Autodesk Inventor part; units mm, degrees
(part 2 of 2)
  line L899 (32.6279, -72.4956) -> (36.6693, -72.5044)
  line L900 (30.5996, -75.9912) -> (32.6279, -72.4956)
  line L901 (32.6127, -79.4956) -> (30.5996, -75.9912)
  line L902 (36.6541, -79.5044) -> (32.6127, -79.4956)
  line L903 (-30.5996, 19.9912) -> (-32.6279, 16.4956)
  line L904 (-32.6127, 23.4956) -> (-30.5996, 19.9912)
  line L905 (-36.6541, 23.5044) -> (-32.6127, 23.4956)
  line L906 (-38.6825, 20.0088) -> (-36.6541, 23.5044)
  line L907 (-36.6693, 16.5044) -> (-38.6825, 20.0088)
  line L908 (-32.6279, 16.4956) -> (-36.6693, 16.5044)
  line L909 (-30.5996, 27.9912) -> (-32.6279, 24.4956)
  line L910 (-32.6127, 31.4956) -> (-30.5996, 27.9912)
  line L911 (-36.6541, 31.5044) -> (-32.6127, 31.4956)
  line L912 (-38.6825, 28.0088) -> (-36.6541, 31.5044)
  line L913 (-36.6693, 24.5044) -> (-38.6825, 28.0088)
  line L914 (-32.6279, 24.4956) -> (-36.6693, 24.5044)
  line L915 (-30.5996, 11.9912) -> (-32.6279, 8.4956)
  line L916 (-32.6127, 15.4956) -> (-30.5996, 11.9912)
  line L917 (-36.6541, 15.5044) -> (-32.6127, 15.4956)
  line L918 (-38.6825, 12.0088) -> (-36.6541, 15.5044)
  line L919 (-36.6693, 8.5044) -> (-38.6825, 12.0088)
  line L920 (-32.6279, 8.4956) -> (-36.6693, 8.5044)
  line L921 (-30.5996, 35.9912) -> (-32.6279, 32.4956)
  line L922 (-32.6127, 39.4956) -> (-30.5996, 35.9912)
  line L923 (-36.6541, 39.5044) -> (-32.6127, 39.4956)
  line L924 (-38.6825, 36.0088) -> (-36.6541, 39.5044)
  line L925 (-36.6693, 32.5044) -> (-38.6825, 36.0088)
  line L926 (-32.6279, 32.4956) -> (-36.6693, 32.5044)
  line L927 (-30.5996, 3.9912) -> (-32.6279, 0.4956)
  line L928 (-32.6127, 7.4956) -> (-30.5996, 3.9912)
  line L929 (-36.6541, 7.5044) -> (-32.6127, 7.4956)
  line L930 (-38.6825, 4.0088) -> (-36.6541, 7.5044)
  line L931 (-36.6693, 0.5044) -> (-38.6825, 4.0088)
  line L932 (-32.6279, 0.4956) -> (-36.6693, 0.5044)
  line L933 (-30.5996, 43.9912) -> (-32.6279, 40.4956)
  line L934 (-32.6127, 47.4956) -> (-30.5996, 43.9912)
  line L935 (-36.6541, 47.5044) -> (-32.6127, 47.4956)
  line L936 (-38.6825, 44.0088) -> (-36.6541, 47.5044)
  line L937 (-36.6693, 40.5044) -> (-38.6825, 44.0088)
  line L938 (-32.6279, 40.4956) -> (-36.6693, 40.5044)
  line L939 (-30.5996, -4.0088) -> (-32.6279, -7.5044)
  line L940 (-32.6127, -0.5044) -> (-30.5996, -4.0088)
  line L941 (-36.6541, -0.4956) -> (-32.6127, -0.5044)
  line L942 (-38.6825, -3.9912) -> (-36.6541, -0.4956)
  line L943 (-36.6693, -7.4956) -> (-38.6825, -3.9912)
  line L944 (-32.6279, -7.5044) -> (-36.6693, -7.4956)
  line L945 (-30.5996, 51.9912) -> (-32.6279, 48.4956)
  line L946 (-32.6127, 55.4956) -> (-30.5996, 51.9912)
  line L947 (-36.6541, 55.5044) -> (-32.6127, 55.4956)
  line L948 (-38.6825, 52.0088) -> (-36.6541, 55.5044)
  line L949 (-36.6693, 48.5044) -> (-38.6825, 52.0088)
  line L950 (-32.6279, 48.4956) -> (-36.6693, 48.5044)
  line L951 (-30.5996, -12.0088) -> (-32.6279, -15.5044)
  line L952 (-32.6127, -8.5044) -> (-30.5996, -12.0088)
  line L953 (-36.6541, -8.4956) -> (-32.6127, -8.5044)
  line L954 (-38.6825, -11.9912) -> (-36.6541, -8.4956)
  line L955 (-36.6693, -15.4956) -> (-38.6825, -11.9912)
  line L956 (-32.6279, -15.5044) -> (-36.6693, -15.4956)
  line L957 (-30.5996, 59.9912) -> (-32.6279, 56.4956)
  line L958 (-32.6127, 63.4956) -> (-30.5996, 59.9912)
  line L959 (-36.6541, 63.5044) -> (-32.6127, 63.4956)
  line L960 (-38.6825, 60.0088) -> (-36.6541, 63.5044)
  line L961 (-36.6693, 56.5044) -> (-38.6825, 60.0088)
  line L962 (-32.6279, 56.4956) -> (-36.6693, 56.5044)
  line L963 (-30.5996, -20.0088) -> (-32.6279, -23.5044)
  line L964 (-32.6127, -16.5044) -> (-30.5996, -20.0088)
  line L965 (-36.6541, -16.4956) -> (-32.6127, -16.5044)
  line L966 (-38.6825, -19.9912) -> (-36.6541, -16.4956)
  line L967 (-36.6693, -23.4956) -> (-38.6825, -19.9912)
  line L968 (-32.6279, -23.5044) -> (-36.6693, -23.4956)
  line L969 (-30.5996, 67.9912) -> (-32.6279, 64.4956)
  line L970 (-32.6127, 71.4956) -> (-30.5996, 67.9912)
  line L971 (-36.6541, 71.5044) -> (-32.6127, 71.4956)
  line L972 (-38.6825, 68.0088) -> (-36.6541, 71.5044)
  line L973 (-36.6693, 64.5044) -> (-38.6825, 68.0088)
  line L974 (-32.6279, 64.4956) -> (-36.6693, 64.5044)
  line L975 (-30.5996, -28.0088) -> (-32.6279, -31.5044)
  line L976 (-32.6127, -24.5044) -> (-30.5996, -28.0088)
  line L977 (-36.6541, -24.4956) -> (-32.6127, -24.5044)
  line L978 (-38.6825, -27.9912) -> (-36.6541, -24.4956)
  line L979 (-36.6693, -31.4956) -> (-38.6825, -27.9912)
  line L980 (-32.6279, -31.5044) -> (-36.6693, -31.4956)
  line L981 (-30.5996, 75.9912) -> (-32.6279, 72.4956)
  line L982 (-32.6127, 79.4956) -> (-30.5996, 75.9912)
  line L983 (-36.6541, 79.5044) -> (-32.6127, 79.4956)
  line L984 (-38.6825, 76.0088) -> (-36.6541, 79.5044)
  line L985 (-36.6693, 72.5044) -> (-38.6825, 76.0088)
  line L986 (-32.6279, 72.4956) -> (-36.6693, 72.5044)
  line L987 (-30.5996, -36.0088) -> (-32.6279, -39.5044)
  line L988 (-32.6127, -32.5044) -> (-30.5996, -36.0088)
  line L989 (-36.6541, -32.4956) -> (-32.6127, -32.5044)
  line L990 (-38.6825, -35.9912) -> (-36.6541, -32.4956)
  line L991 (-36.6693, -39.4956) -> (-38.6825, -35.9912)
  line L992 (-32.6279, -39.5044) -> (-36.6693, -39.4956)
  line L993 (45.6107, -24.0088) -> (43.5823, -27.5044)
  line L994 (43.5975, -20.5044) -> (45.6107, -24.0088)
  line L995 (39.5561, -20.4956) -> (43.5975, -20.5044)
  line L996 (37.5278, -23.9912) -> (39.5561, -20.4956)
  line L997 (39.5409, -27.4956) -> (37.5278, -23.9912)
  line L998 (43.5823, -27.5044) -> (39.5409, -27.4956) construction
  line L999 (45.6107, -16.0088) -> (43.5823, -19.5044)
  line L1000 (43.5975, -12.5044) -> (45.6107, -16.0088)
  line L1001 (39.5561, -12.4956) -> (43.5975, -12.5044)
  line L1002 (37.5278, -15.9912) -> (39.5561, -12.4956)
  line L1003 (39.5409, -19.4956) -> (37.5278, -15.9912)
  line L1004 (43.5823, -19.5044) -> (39.5409, -19.4956)
  line L1005 (45.6107, -32.0088) -> (43.5823, -35.5044)
  line L1006 (43.5975, -28.5044) -> (45.6107, -32.0088)
  line L1007 (39.5561, -28.4956) -> (43.5975, -28.5044)
  line L1008 (37.5278, -31.9912) -> (39.5561, -28.4956)
  line L1009 (39.5409, -35.4956) -> (37.5278, -31.9912)
  line L1010 (43.5823, -35.5044) -> (39.5409, -35.4956)
  line L1011 (45.6107, -8.0088) -> (43.5823, -11.5044)
  line L1012 (43.5975, -4.5044) -> (45.6107, -8.0088)
  line L1013 (39.5561, -4.4956) -> (43.5975, -4.5044)
  line L1014 (37.5278, -7.9912) -> (39.5561, -4.4956)
  line L1015 (39.5409, -11.4956) -> (37.5278, -7.9912)
  line L1016 (43.5823, -11.5044) -> (39.5409, -11.4956)
  line L1017 (45.6107, -40.0088) -> (43.5823, -43.5044)
  line L1018 (43.5975, -36.5044) -> (45.6107, -40.0088)
  line L1019 (39.5561, -36.4956) -> (43.5975, -36.5044)
  line L1020 (37.5278, -39.9912) -> (39.5561, -36.4956)
  line L1021 (39.5409, -43.4956) -> (37.5278, -39.9912)
  line L1022 (43.5823, -43.5044) -> (39.5409, -43.4956)
  line L1023 (45.6107, -0.0088) -> (43.5823, -3.5044)
  line L1024 (43.5975, 3.4956) -> (45.6107, -0.0088)
  line L1025 (39.5561, 3.5044) -> (43.5975, 3.4956)
  line L1026 (37.5278, 0.0088) -> (39.5561, 3.5044)
  line L1027 (39.5409, -3.4956) -> (37.5278, 0.0088)
  line L1028 (43.5823, -3.5044) -> (39.5409, -3.4956)
  line L1029 (45.6107, -48.0088) -> (43.5823, -51.5044)
  line L1030 (43.5975, -44.5044) -> (45.6107, -48.0088)
  line L1031 (39.5561, -44.4956) -> (43.5975, -44.5044)
  line L1032 (37.5278, -47.9912) -> (39.5561, -44.4956)
  line L1033 (39.5409, -51.4956) -> (37.5278, -47.9912)
  line L1034 (43.5823, -51.5044) -> (39.5409, -51.4956)
  line L1035 (45.6107, 7.9912) -> (43.5823, 4.4956)
  line L1036 (43.5975, 11.4956) -> (45.6107, 7.9912)
  line L1037 (39.5561, 11.5044) -> (43.5975, 11.4956)
  line L1038 (37.5278, 8.0088) -> (39.5561, 11.5044)
  line L1039 (39.5409, 4.5044) -> (37.5278, 8.0088)
  line L1040 (43.5823, 4.4956) -> (39.5409, 4.5044)
  line L1041 (45.6107, -56.0088) -> (43.5823, -59.5044)
  line L1042 (43.5975, -52.5044) -> (45.6107, -56.0088)
  line L1043 (39.5561, -52.4956) -> (43.5975, -52.5044)
  line L1044 (37.5278, -55.9912) -> (39.5561, -52.4956)
  line L1045 (39.5409, -59.4956) -> (37.5278, -55.9912)
  line L1046 (43.5823, -59.5044) -> (39.5409, -59.4956)
  line L1047 (45.6107, 15.9912) -> (43.5823, 12.4956)
  line L1048 (43.5975, 19.4956) -> (45.6107, 15.9912)
  line L1049 (39.5561, 19.5044) -> (43.5975, 19.4956)
  line L1050 (37.5278, 16.0088) -> (39.5561, 19.5044)
  line L1051 (39.5409, 12.5044) -> (37.5278, 16.0088)
  line L1052 (43.5823, 12.4956) -> (39.5409, 12.5044)
  line L1053 (45.6107, -64.0088) -> (43.5823, -67.5044)
  line L1054 (43.5975, -60.5044) -> (45.6107, -64.0088)
  line L1055 (39.5561, -60.4956) -> (43.5975, -60.5044)
  line L1056 (37.5278, -63.9912) -> (39.5561, -60.4956)
  line L1057 (39.5409, -67.4956) -> (37.5278, -63.9912)
  line L1058 (43.5823, -67.5044) -> (39.5409, -67.4956)
  line L1059 (45.6107, 23.9912) -> (43.5823, 20.4956)
  line L1060 (43.5975, 27.4956) -> (45.6107, 23.9912)
  line L1061 (39.5561, 27.5044) -> (43.5975, 27.4956)
  line L1062 (37.5278, 24.0088) -> (39.5561, 27.5044)
  line L1063 (39.5409, 20.5044) -> (37.5278, 24.0088)
  line L1064 (43.5823, 20.4956) -> (39.5409, 20.5044)
  line L1065 (45.6107, -72.0088) -> (43.5823, -75.5044)
  line L1066 (43.5975, -68.5044) -> (45.6107, -72.0088)
  line L1067 (39.5561, -68.4956) -> (43.5975, -68.5044)
  line L1068 (37.5278, -71.9912) -> (39.5561, -68.4956)
  line L1069 (39.5409, -75.4956) -> (37.5278, -71.9912)
  line L1070 (43.5823, -75.5044) -> (39.5409, -75.4956)
  line L1071 (45.6107, 31.9912) -> (43.5823, 28.4956)
  line L1072 (43.5975, 35.4956) -> (45.6107, 31.9912)
  line L1073 (39.5561, 35.5044) -> (43.5975, 35.4956)
  line L1074 (37.5278, 32.0088) -> (39.5561, 35.5044)
  line L1075 (39.5409, 28.5044) -> (37.5278, 32.0088)
  line L1076 (43.5823, 28.4956) -> (39.5409, 28.5044)
  line L1077 (45.6107, -80.0088) -> (43.5823, -83.5044)
  line L1078 (43.5975, -76.5044) -> (45.6107, -80.0088)
  line L1079 (39.5561, -76.4956) -> (43.5975, -76.5044)
  line L1080 (37.5278, -79.9912) -> (39.5561, -76.4956)
  line L1081 (39.5409, -83.4956) -> (37.5278, -79.9912)
  line L1082 (43.5823, -83.5044) -> (39.5409, -83.4956)
  line L1083 (-37.5278, 23.9912) -> (-39.5561, 20.4956)
  line L1084 (-39.5409, 27.4956) -> (-37.5278, 23.9912)
  line L1085 (-43.5823, 27.5044) -> (-39.5409, 27.4956)
  line L1086 (-45.6107, 24.0088) -> (-43.5823, 27.5044)
  line L1087 (-43.5975, 20.5044) -> (-45.6107, 24.0088)
  line L1088 (-39.5561, 20.4956) -> (-43.5975, 20.5044)
  line L1089 (-37.5278, 31.9912) -> (-39.5561, 28.4956)
  line L1090 (-39.5409, 35.4956) -> (-37.5278, 31.9912)
  line L1091 (-43.5823, 35.5044) -> (-39.5409, 35.4956)
  line L1092 (-45.6107, 32.0088) -> (-43.5823, 35.5044)
  line L1093 (-43.5975, 28.5044) -> (-45.6107, 32.0088)
  line L1094 (-39.5561, 28.4956) -> (-43.5975, 28.5044)
  line L1095 (-37.5278, 15.9912) -> (-39.5561, 12.4956)
  line L1096 (-39.5409, 19.4956) -> (-37.5278, 15.9912)
  line L1097 (-43.5823, 19.5044) -> (-39.5409, 19.4956)
  line L1098 (-45.6107, 16.0088) -> (-43.5823, 19.5044)
  line L1099 (-43.5975, 12.5044) -> (-45.6107, 16.0088)
  line L1100 (-39.5561, 12.4956) -> (-43.5975, 12.5044)
  line L1101 (-37.5278, 39.9912) -> (-39.5561, 36.4956)
  line L1102 (-39.5409, 43.4956) -> (-37.5278, 39.9912)
  line L1103 (-43.5823, 43.5044) -> (-39.5409, 43.4956)
  line L1104 (-45.6107, 40.0088) -> (-43.5823, 43.5044)
  line L1105 (-43.5975, 36.5044) -> (-45.6107, 40.0088)
  line L1106 (-39.5561, 36.4956) -> (-43.5975, 36.5044)
  line L1107 (-37.5278, 7.9912) -> (-39.5561, 4.4956)
  line L1108 (-39.5409, 11.4956) -> (-37.5278, 7.9912)
  line L1109 (-43.5823, 11.5044) -> (-39.5409, 11.4956)
  line L1110 (-45.6107, 8.0088) -> (-43.5823, 11.5044)
  line L1111 (-43.5975, 4.5044) -> (-45.6107, 8.0088)
  line L1112 (-39.5561, 4.4956) -> (-43.5975, 4.5044)
  line L1113 (-37.5278, 47.9912) -> (-39.5561, 44.4956)
  line L1114 (-39.5409, 51.4956) -> (-37.5278, 47.9912)
  line L1115 (-43.5823, 51.5044) -> (-39.5409, 51.4956)
  line L1116 (-45.6107, 48.0088) -> (-43.5823, 51.5044)
  line L1117 (-43.5975, 44.5044) -> (-45.6107, 48.0088)
  line L1118 (-39.5561, 44.4956) -> (-43.5975, 44.5044)
  line L1119 (-37.5278, -0.0088) -> (-39.5561, -3.5044)
  line L1120 (-39.5409, 3.4956) -> (-37.5278, -0.0088)
  line L1121 (-43.5823, 3.5044) -> (-39.5409, 3.4956)
  line L1122 (-45.6107, 0.0088) -> (-43.5823, 3.5044)
  line L1123 (-43.5975, -3.4956) -> (-45.6107, 0.0088)
  line L1124 (-39.5561, -3.5044) -> (-43.5975, -3.4956)
  line L1125 (-37.5278, 55.9912) -> (-39.5561, 52.4956)
  line L1126 (-39.5409, 59.4956) -> (-37.5278, 55.9912)
  line L1127 (-43.5823, 59.5044) -> (-39.5409, 59.4956)
  line L1128 (-45.6107, 56.0088) -> (-43.5823, 59.5044)
  line L1129 (-43.5975, 52.5044) -> (-45.6107, 56.0088)
  line L1130 (-39.5561, 52.4956) -> (-43.5975, 52.5044)
  line L1131 (-37.5278, -8.0088) -> (-39.5561, -11.5044)
  line L1132 (-39.5409, -4.5044) -> (-37.5278, -8.0088)
  line L1133 (-43.5823, -4.4956) -> (-39.5409, -4.5044)
  line L1134 (-45.6107, -7.9912) -> (-43.5823, -4.4956)
  line L1135 (-43.5975, -11.4956) -> (-45.6107, -7.9912)
  line L1136 (-39.5561, -11.5044) -> (-43.5975, -11.4956)
  line L1137 (-37.5278, 63.9912) -> (-39.5561, 60.4956)
  line L1138 (-39.5409, 67.4956) -> (-37.5278, 63.9912)
  line L1139 (-43.5823, 67.5044) -> (-39.5409, 67.4956)
  line L1140 (-45.6107, 64.0088) -> (-43.5823, 67.5044)
  line L1141 (-43.5975, 60.5044) -> (-45.6107, 64.0088)
  line L1142 (-39.5561, 60.4956) -> (-43.5975, 60.5044)
  line L1143 (-37.5278, -16.0088) -> (-39.5561, -19.5044)
  line L1144 (-39.5409, -12.5044) -> (-37.5278, -16.0088)
  line L1145 (-43.5823, -12.4956) -> (-39.5409, -12.5044)
  line L1146 (-45.6107, -15.9912) -> (-43.5823, -12.4956)
  line L1147 (-43.5975, -19.4956) -> (-45.6107, -15.9912)
  line L1148 (-39.5561, -19.5044) -> (-43.5975, -19.4956)
  line L1149 (-37.5278, 71.9912) -> (-39.5561, 68.4956)
  line L1150 (-39.5409, 75.4956) -> (-37.5278, 71.9912)
  line L1151 (-43.5823, 75.5044) -> (-39.5409, 75.4956)
  line L1152 (-45.6107, 72.0088) -> (-43.5823, 75.5044)
  line L1153 (-43.5975, 68.5044) -> (-45.6107, 72.0088)
  line L1154 (-39.5561, 68.4956) -> (-43.5975, 68.5044)
  line L1155 (-37.5278, -24.0088) -> (-39.5561, -27.5044)
  line L1156 (-39.5409, -20.5044) -> (-37.5278, -24.0088)
  line L1157 (-43.5823, -20.4956) -> (-39.5409, -20.5044)
  line L1158 (-45.6107, -23.9912) -> (-43.5823, -20.4956)
  line L1159 (-43.5975, -27.4956) -> (-45.6107, -23.9912)
  line L1160 (-39.5561, -27.5044) -> (-43.5975, -27.4956)
  line L1161 (-37.5278, 79.9912) -> (-39.5561, 76.4956)
  line L1162 (-39.5409, 83.4956) -> (-37.5278, 79.9912)
  line L1163 (-43.5823, 83.5044) -> (-39.5409, 83.4956)
  line L1164 (-45.6107, 80.0088) -> (-43.5823, 83.5044)
  line L1165 (-43.5975, 76.5044) -> (-45.6107, 80.0088)
  line L1166 (-39.5561, 76.4956) -> (-43.5975, 76.5044)
  line L1167 (-37.5278, -32.0088) -> (-39.5561, -35.5044)
  line L1168 (-39.5409, -28.5044) -> (-37.5278, -32.0088)
  line L1169 (-43.5823, -28.4956) -> (-39.5409, -28.5044)
  line L1170 (-45.6107, -31.9912) -> (-43.5823, -28.4956)
  line L1171 (-43.5975, -35.4956) -> (-45.6107, -31.9912)
  line L1172 (-39.5561, -35.5044) -> (-43.5975, -35.4956)
  line L1173 (52.5389, -28.0088) -> (50.5105, -31.5044)
  line L1174 (50.5257, -24.5044) -> (52.5389, -28.0088)
  line L1175 (46.4843, -24.4956) -> (50.5257, -24.5044)
  line L1176 (44.456, -27.9912) -> (46.4843, -24.4956)
  line L1177 (46.4691, -31.4956) -> (44.456, -27.9912)
  line L1178 (50.5105, -31.5044) -> (46.4691, -31.4956)
  line L1179 (52.5389, -20.0088) -> (50.5105, -23.5044) construction
  line L1180 (50.5257, -16.5044) -> (52.5389, -20.0088) construction
  line L1181 (46.4843, -16.4956) -> (50.5257, -16.5044)
  line L1182 (44.456, -19.9912) -> (46.4843, -16.4956)
  line L1183 (46.4691, -23.4956) -> (44.456, -19.9912)
  line L1184 (50.5105, -23.5044) -> (46.4691, -23.4956)
  line L1185 (52.5389, -36.0088) -> (50.5105, -39.5044)
  line L1186 (50.5257, -32.5044) -> (52.5389, -36.0088)
  line L1187 (46.4843, -32.4956) -> (50.5257, -32.5044)
  line L1188 (44.456, -35.9912) -> (46.4843, -32.4956)
  line L1189 (46.4691, -39.4956) -> (44.456, -35.9912)
  line L1190 (50.5105, -39.5044) -> (46.4691, -39.4956)
  line L1191 (52.5389, -12.0088) -> (50.5105, -15.5044)
  line L1192 (50.5257, -8.5044) -> (52.5389, -12.0088)
  line L1193 (46.4843, -8.4956) -> (50.5257, -8.5044)
  line L1194 (44.456, -11.9912) -> (46.4843, -8.4956)
  line L1195 (46.4691, -15.4956) -> (44.456, -11.9912)
  line L1196 (50.5105, -15.5044) -> (46.4691, -15.4956)
  line L1197 (52.5389, -44.0088) -> (50.5105, -47.5044)
  line L1198 (50.5257, -40.5044) -> (52.5389, -44.0088)
  line L1199 (46.4843, -40.4956) -> (50.5257, -40.5044)
  line L1200 (44.456, -43.9912) -> (46.4843, -40.4956)
  line L1201 (46.4691, -47.4956) -> (44.456, -43.9912)
  line L1202 (50.5105, -47.5044) -> (46.4691, -47.4956)
  line L1203 (52.5389, -4.0088) -> (50.5105, -7.5044)
  line L1204 (50.5257, -0.5044) -> (52.5389, -4.0088)
  line L1205 (46.4843, -0.4956) -> (50.5257, -0.5044)
  line L1206 (44.456, -3.9912) -> (46.4843, -0.4956)
  line L1207 (46.4691, -7.4956) -> (44.456, -3.9912)
  line L1208 (50.5105, -7.5044) -> (46.4691, -7.4956)
  line L1209 (52.5389, -52.0088) -> (50.5105, -55.5044)
  line L1210 (50.5257, -48.5044) -> (52.5389, -52.0088)
  line L1211 (46.4843, -48.4956) -> (50.5257, -48.5044)
  line L1212 (44.456, -51.9912) -> (46.4843, -48.4956)
  line L1213 (46.4691, -55.4956) -> (44.456, -51.9912)
  line L1214 (50.5105, -55.5044) -> (46.4691, -55.4956)
  line L1215 (52.5389, 3.9912) -> (50.5105, 0.4956)
  line L1216 (50.5257, 7.4956) -> (52.5389, 3.9912)
  line L1217 (46.4843, 7.5044) -> (50.5257, 7.4956)
  line L1218 (44.456, 4.0088) -> (46.4843, 7.5044)
  line L1219 (46.4691, 0.5044) -> (44.456, 4.0088)
  line L1220 (50.5105, 0.4956) -> (46.4691, 0.5044)
  line L1221 (52.5389, -60.0088) -> (50.5105, -63.5044)
  line L1222 (50.5257, -56.5044) -> (52.5389, -60.0088)
  line L1223 (46.4843, -56.4956) -> (50.5257, -56.5044)
  line L1224 (44.456, -59.9912) -> (46.4843, -56.4956)
  line L1225 (46.4691, -63.4956) -> (44.456, -59.9912)
  line L1226 (50.5105, -63.5044) -> (46.4691, -63.4956)
  line L1227 (52.5389, 11.9912) -> (50.5105, 8.4956)
  line L1228 (50.5257, 15.4956) -> (52.5389, 11.9912)
  line L1229 (46.4843, 15.5044) -> (50.5257, 15.4956)
  line L1230 (44.456, 12.0088) -> (46.4843, 15.5044)
  line L1231 (46.4691, 8.5044) -> (44.456, 12.0088)
  line L1232 (50.5105, 8.4956) -> (46.4691, 8.5044)
  line L1233 (52.5389, -68.0088) -> (50.5105, -71.5044)
  line L1234 (50.5257, -64.5044) -> (52.5389, -68.0088)
  line L1235 (46.4843, -64.4956) -> (50.5257, -64.5044)
  line L1236 (44.456, -67.9912) -> (46.4843, -64.4956)
  line L1237 (46.4691, -71.4956) -> (44.456, -67.9912)
  line L1238 (50.5105, -71.5044) -> (46.4691, -71.4956)
  line L1239 (52.5389, 19.9912) -> (50.5105, 16.4956)
  line L1240 (50.5257, 23.4956) -> (52.5389, 19.9912)
  line L1241 (46.4843, 23.5044) -> (50.5257, 23.4956)
  line L1242 (44.456, 20.0088) -> (46.4843, 23.5044)
  line L1243 (46.4691, 16.5044) -> (44.456, 20.0088)
  line L1244 (50.5105, 16.4956) -> (46.4691, 16.5044)
  line L1245 (52.5389, -76.0088) -> (50.5105, -79.5044)
  line L1246 (50.5257, -72.5044) -> (52.5389, -76.0088)
  line L1247 (46.4843, -72.4956) -> (50.5257, -72.5044)
  line L1248 (44.456, -75.9912) -> (46.4843, -72.4956)
  line L1249 (46.4691, -79.4956) -> (44.456, -75.9912)
  line L1250 (50.5105, -79.5044) -> (46.4691, -79.4956)
  line L1251 (52.5389, 27.9912) -> (50.5105, 24.4956)
  line L1252 (50.5257, 31.4956) -> (52.5389, 27.9912)
  line L1253 (46.4843, 31.5044) -> (50.5257, 31.4956)
  line L1254 (44.456, 28.0088) -> (46.4843, 31.5044)
  line L1255 (46.4691, 24.5044) -> (44.456, 28.0088)
  line L1256 (50.5105, 24.4956) -> (46.4691, 24.5044)
  line L1257 (52.5389, -84.0088) -> (50.5105, -87.5044)
  line L1258 (50.5257, -80.5044) -> (52.5389, -84.0088)
  line L1259 (46.4843, -80.4956) -> (50.5257, -80.5044)
  line L1260 (44.456, -83.9912) -> (46.4843, -80.4956)
  line L1261 (46.4691, -87.4956) -> (44.456, -83.9912)
  line L1262 (50.5105, -87.5044) -> (46.4691, -87.4956)
  line L1263 (-44.456, 27.9912) -> (-46.4843, 24.4956)
  line L1264 (-46.4691, 31.4956) -> (-44.456, 27.9912)
  line L1265 (-50.5105, 31.5044) -> (-46.4691, 31.4956)
  line L1266 (-52.5389, 28.0088) -> (-50.5105, 31.5044)
  line L1267 (-50.5257, 24.5044) -> (-52.5389, 28.0088)
  line L1268 (-46.4843, 24.4956) -> (-50.5257, 24.5044)
  line L1269 (-44.456, 35.9912) -> (-46.4843, 32.4956)
  line L1270 (-46.4691, 39.4956) -> (-44.456, 35.9912)
  line L1271 (-50.5105, 39.5044) -> (-46.4691, 39.4956)
  line L1272 (-52.5389, 36.0088) -> (-50.5105, 39.5044)
  line L1273 (-50.5257, 32.5044) -> (-52.5389, 36.0088)
  line L1274 (-46.4843, 32.4956) -> (-50.5257, 32.5044)
  line L1275 (-44.456, 19.9912) -> (-46.4843, 16.4956)
  line L1276 (-46.4691, 23.4956) -> (-44.456, 19.9912)
  line L1277 (-50.5105, 23.5044) -> (-46.4691, 23.4956)
  line L1278 (-52.5389, 20.0088) -> (-50.5105, 23.5044)
  line L1279 (-50.5257, 16.5044) -> (-52.5389, 20.0088)
  line L1280 (-46.4843, 16.4956) -> (-50.5257, 16.5044)
  line L1281 (-44.456, 43.9912) -> (-46.4843, 40.4956)
  line L1282 (-46.4691, 47.4956) -> (-44.456, 43.9912)
  line L1283 (-50.5105, 47.5044) -> (-46.4691, 47.4956)
  line L1284 (-52.5389, 44.0088) -> (-50.5105, 47.5044)
  line L1285 (-50.5257, 40.5044) -> (-52.5389, 44.0088)
  line L1286 (-46.4843, 40.4956) -> (-50.5257, 40.5044)
  line L1287 (-44.456, 11.9912) -> (-46.4843, 8.4956)
  line L1288 (-46.4691, 15.4956) -> (-44.456, 11.9912)
  line L1289 (-50.5105, 15.5044) -> (-46.4691, 15.4956)
  line L1290 (-52.5389, 12.0088) -> (-50.5105, 15.5044)
  line L1291 (-50.5257, 8.5044) -> (-52.5389, 12.0088)
  line L1292 (-46.4843, 8.4956) -> (-50.5257, 8.5044)
  line L1293 (-44.456, 51.9912) -> (-46.4843, 48.4956)
  line L1294 (-46.4691, 55.4956) -> (-44.456, 51.9912)
  line L1295 (-50.5105, 55.5044) -> (-46.4691, 55.4956)
  line L1296 (-52.5389, 52.0088) -> (-50.5105, 55.5044)
  line L1297 (-50.5257, 48.5044) -> (-52.5389, 52.0088)
  line L1298 (-46.4843, 48.4956) -> (-50.5257, 48.5044)
  line L1299 (-44.456, 3.9912) -> (-46.4843, 0.4956)
  line L1300 (-46.4691, 7.4956) -> (-44.456, 3.9912)
  line L1301 (-50.5105, 7.5044) -> (-46.4691, 7.4956)
  line L1302 (-52.5389, 4.0088) -> (-50.5105, 7.5044)
  line L1303 (-50.5257, 0.5044) -> (-52.5389, 4.0088)
  line L1304 (-46.4843, 0.4956) -> (-50.5257, 0.5044)
  line L1305 (-44.456, 59.9912) -> (-46.4843, 56.4956)
  line L1306 (-46.4691, 63.4956) -> (-44.456, 59.9912)
  line L1307 (-50.5105, 63.5044) -> (-46.4691, 63.4956)
  line L1308 (-52.5389, 60.0088) -> (-50.5105, 63.5044)
  line L1309 (-50.5257, 56.5044) -> (-52.5389, 60.0088)
  line L1310 (-46.4843, 56.4956) -> (-50.5257, 56.5044)
  line L1311 (-44.456, -4.0088) -> (-46.4843, -7.5044)
  line L1312 (-46.4691, -0.5044) -> (-44.456, -4.0088)
  line L1313 (-50.5105, -0.4956) -> (-46.4691, -0.5044)
  line L1314 (-52.5389, -3.9912) -> (-50.5105, -0.4956)
  line L1315 (-50.5257, -7.4956) -> (-52.5389, -3.9912)
  line L1316 (-46.4843, -7.5044) -> (-50.5257, -7.4956)
  line L1317 (-44.456, 67.9912) -> (-46.4843, 64.4956)
  line L1318 (-46.4691, 71.4956) -> (-44.456, 67.9912)
  line L1319 (-50.5105, 71.5044) -> (-46.4691, 71.4956)
  line L1320 (-52.5389, 68.0088) -> (-50.5105, 71.5044)
  line L1321 (-50.5257, 64.5044) -> (-52.5389, 68.0088)
  line L1322 (-46.4843, 64.4956) -> (-50.5257, 64.5044)
  line L1323 (-44.456, -12.0088) -> (-46.4843, -15.5044)
  line L1324 (-46.4691, -8.5044) -> (-44.456, -12.0088)
  line L1325 (-50.5105, -8.4956) -> (-46.4691, -8.5044)
  line L1326 (-52.5389, -11.9912) -> (-50.5105, -8.4956)
  line L1327 (-50.5257, -15.4956) -> (-52.5389, -11.9912)
  line L1328 (-46.4843, -15.5044) -> (-50.5257, -15.4956)
  line L1329 (-44.456, 75.9912) -> (-46.4843, 72.4956)
  line L1330 (-46.4691, 79.4956) -> (-44.456, 75.9912)
  line L1331 (-50.5105, 79.5044) -> (-46.4691, 79.4956)
  line L1332 (-52.5389, 76.0088) -> (-50.5105, 79.5044)
  line L1333 (-50.5257, 72.5044) -> (-52.5389, 76.0088)
  line L1334 (-46.4843, 72.4956) -> (-50.5257, 72.5044)
  line L1335 (-44.456, -20.0088) -> (-46.4843, -23.5044)
  line L1336 (-46.4691, -16.5044) -> (-44.456, -20.0088)
  line L1337 (-50.5105, -16.4956) -> (-46.4691, -16.5044)
  line L1338 (-52.5389, -19.9912) -> (-50.5105, -16.4956)
  line L1339 (-50.5257, -23.4956) -> (-52.5389, -19.9912)
  line L1340 (-46.4843, -23.5044) -> (-50.5257, -23.4956)
  line L1341 (-44.456, 83.9912) -> (-46.4843, 80.4956)
  line L1342 (-46.4691, 87.4956) -> (-44.456, 83.9912)
  line L1343 (-50.5105, 87.5044) -> (-46.4691, 87.4956)
  line L1344 (-52.5389, 84.0088) -> (-50.5105, 87.5044)
  line L1345 (-50.5257, 80.5044) -> (-52.5389, 84.0088)
  line L1346 (-46.4843, 80.4956) -> (-50.5257, 80.5044)
  line L1347 (-44.456, -28.0088) -> (-46.4843, -31.5044)
  line L1348 (-46.4691, -24.5044) -> (-44.456, -28.0088)
  line L1349 (-50.5105, -24.4956) -> (-46.4691, -24.5044)
  line L1350 (-52.5389, -27.9912) -> (-50.5105, -24.4956)
  line L1351 (-50.5257, -31.4956) -> (-52.5389, -27.9912)
  line L1352 (-46.4843, -31.5044) -> (-50.5257, -31.4956)
  circle A0 centre (0, 0) radius 47.5 projected
  circle A1 centre (0, 0) radius 46.5
  line L1353 (30.5996, 36.0088) -> (32.6127, 32.5044)
  line L1354 (32.6127, 32.5044) -> (36.6541, 32.4956)
  line L1355 (30.5996, 36.0088) -> (32.6279, 39.5044)
  line L1356 (46.4843, 15.5044) -> (44.456, 12.0088)
  line L1357 (46.4691, 8.5044) -> (50.5105, 8.4956)
  line L1358 (46.4691, 8.5044) -> (44.456, 12.0088)
  line L1359 (50.5257, -8.5044) -> (46.4843, -8.4956)
  line L1360 (44.456, -11.9912) -> (46.4691, -15.4956)
  line L1361 (46.4843, -8.4956) -> (44.456, -11.9912)
  line L1362 (36.6693, -32.5044) -> (32.6279, -32.4956)
  line L1363 (30.5996, -35.9912) -> (32.6127, -39.4956)
  line L1364 (32.6279, -32.4956) -> (30.5996, -35.9912)
  line L1365 (17.8978, -48.0088) -> (15.8847, -44.5044)
  line L1366 (11.8433, -44.4956) -> (15.8847, -44.5044)
  line L1367 (9.815, -47.9912) -> (11.8281, -51.4956)
  line L1368 (11.8433, -44.4956) -> (9.815, -47.9912)
  line L1369 (-11.8281, -44.5044) -> (-15.8695, -44.4956)
  line L1370 (-17.8978, -47.9912) -> (-15.8695, -44.4956)
  line L1371 (-11.8281, -44.5044) -> (-9.815, -48.0088)
  line L1372 (39.5409, -27.4956) -> (43.5823, -27.5044)
  circle A2 centre (0, 0) radius 52.5 projected
  point P0 (-0.0076, -3.5)
  point P1 (3.0311, 6.25)
  point P2 (0, 11.5)
  point P3 (-0.0076, 4.5)
  point P4 (3.0311, -9.75)
  point P5 (0, -4.5)
  point P6 (-0.0076, -11.5)
  point P7 (3.0311, 14.25)
  point P8 (0, 19.5)
  point P9 (-0.0076, 12.5)
  point P10 (3.0311, -17.75)
  point P11 (0, -12.5)
  point P12 (-0.0076, -19.5)
  point P13 (3.0311, 22.25)
  point P14 (0, 27.5)
  point P15 (-0.0076, 20.5)
  point P16 (3.0311, -25.75)
  point P17 (0, -20.5)
  point P18 (-0.0076, -27.5)
  point P19 (3.0311, 30.25)
  point P20 (0, 35.5)
  point P21 (-0.0076, 28.5)
  point P22 (3.0311, -33.75)
  point P23 (0, -28.5)
  point P24 (-0.0076, -35.5)
  point P25 (3.0311, 38.25)
  point P26 (0, 43.5)
  point P27 (-0.0076, 36.5)
  point P28 (3.0311, -41.75)
  point P29 (0, -36.5)
  point P30 (-0.0076, -43.5)
  point P31 (3.0311, 46.25)
  point P32 (0, 51.5)
  point P33 (-0.0076, 44.5)
  point P34 (3.0311, -49.75)
  point P35 (0, -44.5)
  point P36 (-0.0076, -51.5)
  point P37 (3.0311, 54.25)
  point P38 (0, 59.5)
  point P39 (-0.0076, 52.5)
  point P40 (3.0311, -57.75)
  point P41 (0, -52.5)
  point P42 (-0.0076, -59.5)
  point P43 (9.9593, -5.75)
  point P44 (6.9282, -0.5)
  point P45 (6.9206, -7.5)
  point P46 (9.9593, 2.25)
  point P47 (6.9282, 7.5)
  point P48 (6.9206, 0.5)
  point P49 (9.9593, -13.75)
  point P50 (6.9282, -8.5)
  point P51 (6.9206, -15.5)
  point P52 (9.9593, 10.25)
  point P53 (6.9282, 15.5)
  point P54 (6.9206, 8.5)
  point P55 (9.9593, -21.75)
  point P56 (6.9282, -16.5)
  point P57 (6.9206, -23.5)
  point P58 (9.9593, 18.25)
  point P59 (6.9282, 23.5)
  point P60 (6.9206, 16.5)
  point P61 (9.9593, -29.75)
  point P62 (6.9282, -24.5)
  point P63 (6.9206, -31.5)
  point P64 (9.9593, 26.25)
  point P65 (6.9282, 31.5)
  point P66 (6.9206, 24.5)
  point P67 (9.9593, -37.75)
  point P68 (6.9282, -32.5)
  point P69 (6.9206, -39.5)
  point P70 (9.9593, 34.25)
  point P71 (6.9282, 39.5)
  point P72 (6.9206, 32.5)
  point P73 (9.9593, -45.75)
  point P74 (6.9282, -40.5)
  point P75 (6.9206, -47.5)
  point P76 (9.9593, 42.25)
  point P77 (6.9282, 47.5)
  point P78 (6.9206, 40.5)
  point P79 (9.9593, -53.75)
  point P80 (6.9282, -48.5)
  point P81 (6.9206, -55.5)
  point P82 (9.9593, 50.25)
  point P83 (6.9282, 55.5)
  point P84 (6.9206, 48.5)
  point P85 (9.9593, -61.75)
  point P86 (6.9282, -56.5)
  point P87 (6.9206, -63.5)
  point P88 (-3.8971, 2.25)
  point P89 (-6.9282, 7.5)
  point P90 (-6.9358, 0.5)
  point P91 (-3.8971, 10.25)
  point P92 (-6.9282, 15.5)
  point P93 (-6.9358, 8.5)
  point P94 (-3.8971, -5.75)
  point P95 (-6.9282, -0.5)
  point P96 (-6.9358, -7.5)
  point P97 (-3.8971, 18.25)
  point P98 (-6.9282, 23.5)
  point P99 (-6.9358, 16.5)
  point P100 (-3.8971, -13.75)
  point P101 (-6.9282, -8.5)
  point P102 (-6.9358, -15.5)
  point P103 (-3.8971, 26.25)
  point P104 (-6.9282, 31.5)
  point P105 (-6.9358, 24.5)
  point P106 (-3.8971, -21.75)
  point P107 (-6.9282, -16.5)
  point P108 (-6.9358, -23.5)
  point P109 (-3.8971, 34.25)
  point P110 (-6.9282, 39.5)
  point P111 (-6.9358, 32.5)
  point P112 (-3.8971, -29.75)
  point P113 (-6.9282, -24.5)
  point P114 (-6.9358, -31.5)
  point P115 (-3.8971, 42.25)
  point P116 (-6.9282, 47.5)
  point P117 (-6.9358, 40.5)
  point P118 (-3.8971, -37.75)
  point P119 (-6.9282, -32.5)
  point P120 (-6.9358, -39.5)
  point P121 (-3.8971, 50.25)
  point P122 (-6.9282, 55.5)
  point P123 (-6.9358, 48.5)
  point P124 (-3.8971, -45.75)
  point P125 (-6.9282, -40.5)
  point P126 (-6.9358, -47.5)
  point P127 (-3.8971, 58.25)
  point P128 (-6.9282, 63.5)
  point P129 (-6.9358, 56.5)
  point P130 (-3.8971, -53.75)
  point P131 (-6.9282, -48.5)
  point P132 (-6.9358, -55.5)
  point P133 (16.8875, -9.75)
  point P134 (13.8564, -4.5)
  point P135 (13.8488, -11.5)
  point P136 (16.8875, -1.75)
  point P137 (13.8564, 3.5)
  point P138 (13.8488, -3.5)
  point P139 (16.8875, -17.75)
  point P140 (13.8564, -12.5)
  point P141 (13.8488, -19.5)
  point P142 (16.8875, 6.25)
  point P143 (13.8564, 11.5)
  point P144 (13.8488, 4.5)
  point P145 (16.8875, -25.75)
  point P146 (13.8564, -20.5)
  point P147 (13.8488, -27.5)
  point P148 (16.8875, 14.25)
  point P149 (13.8564, 19.5)
  point P150 (13.8488, 12.5)
  point P151 (16.8875, -33.75)
  point P152 (13.8564, -28.5)
  point P153 (13.8488, -35.5)
  point P154 (16.8875, 22.25)
  point P155 (13.8564, 27.5)
  point P156 (13.8488, 20.5)
  point P157 (16.8875, -41.75)
  point P158 (13.8564, -36.5)
  point P159 (13.8488, -43.5)
  point P160 (16.8875, 30.25)
  point P161 (13.8564, 35.5)
  point P162 (13.8488, 28.5)
  point P163 (16.8875, -49.75)
  point P164 (13.8564, -44.5)
  point P165 (13.8488, -51.5)
  point P166 (16.8875, 38.25)
  point P167 (13.8564, 43.5)
  point P168 (13.8488, 36.5)
  point P169 (16.8875, -57.75)
  point P170 (13.8564, -52.5)
  point P171 (13.8488, -59.5)
  point P172 (16.8875, 46.25)
  point P173 (13.8564, 51.5)
  point P174 (13.8488, 44.5)
  point P175 (16.8875, -65.75)
  point P176 (13.8564, -60.5)
  point P177 (13.8488, -67.5)
  point P178 (-10.8253, 6.25)
  point P179 (-13.8564, 11.5)
  point P180 (-13.864, 4.5)
  point P181 (-10.8253, 14.25)
  point P182 (-13.8564, 19.5)
  point P183 (-13.864, 12.5)
  point P184 (-10.8253, -1.75)
  point P185 (-13.8564, 3.5)
  point P186 (-13.864, -3.5)
  point P187 (-10.8253, 22.25)
  point P188 (-13.8564, 27.5)
  point P189 (-13.864, 20.5)
  point P190 (-10.8253, -9.75)
  point P191 (-13.8564, -4.5)
  point P192 (-13.864, -11.5)
  point P193 (-10.8253, 30.25)
  point P194 (-13.8564, 35.5)
  point P195 (-13.864, 28.5)
  point P196 (-10.8253, -17.75)
  point P197 (-13.8564, -12.5)
  point P198 (-13.864, -19.5)
  point P199 (-10.8253, 38.25)
  dimension "d65" = 7
  dimension "d69" = 8
  dimension "d72" = 8
  constraints: 2746 end point, 450 point on line, 20 equal length, 2 coincident, 1 horizontal, 1 midpoint, 1 perpendicular, 1 vertical, 3376 other
  measures "d65" distance from line of point (-0.008, -3.5) L2
  measures "d69" distance of L3.end L9.start
  measures "d72" distance of L3.end L93.start
extrude "Extrusion10" cut sketch "Sketch14" against normal blind 10 contours L21 L26 L25 L24 L23 L22 | L27 L32 L31 L30 L29 L28 | L33 L38 L37 L36 L35 L34 | L39 L44 L43 L42 L41 L40 | L45 L50 L49 L48 L47 L46 | L51 L56 L55 L54 L53 L52 | L57 L62 L61 L60 L59 L58 | L63 L68 L67 L66 L65 L64 | L69 L74 L73 A1 | A1 L160 L159 L164 L163 L162 | L238 L237 L242 L241 L240 A1 | A1 L356 L355 | L417 L422 A1 | A1 L531 L536 L535 | L585 L590 L589 A1 | A1 L716 L715 L714 | L754 L753 L758 A1 | A1 L896 L895 | L921 L926 A1 | A1 L879 L884 L883 L882 L881 | L911 L910 L909 L914 L913 A1 | A1 L1064 L1063 L1062 | L1084 L1083 L1088 A1 | A1 L1047 L1052 L1051 L1050 L1049 | L1097 L1096 L1095 L1100 L1099 A1 | A1 L1231 L1230 | L1288 L1287 A1 | A1 L1220 L1219 L1218 | L1300 L1299 L1304 A1 | A1 L1207 L1206 L1205 | L1313 L1312 L1311 A1 | A2 L1315 L1314 | A1 L1195 L1194 | L1324 L1323 A1 | A1 L1004 L1003 L1002 L1001 L1000 | L1146 L1145 L1144 L1143 L1148 A1 | A1 L997 L996 L995 | L1157 L1156 L1155 A1 | A1 L830 L829 L828 L827 L826 | L978 L977 L976 L975 L980 A1 | A1 L840 L839 | L989 L988 A1 | A1 L673 L672 L671 | L809 L808 L807 A1 | A1 L504 L503 L502 | L630 L629 L628 A1 | A1 L336 L335 | L449 L448 A1 | A1 L157 L156 L155 L154 L153 | L259 L258 L257 L256 L255 A1 | A1 L78 L77 L76 | L117 L122 L121 L120 L119 L118 | L123 L128 L127 L126 L125 L124 | L129 L134 L133 L132 L131 L130 | L135 L140 L139 L138 L137 L136 | L141 L146 L145 L144 L143 L142 | L147 L152 L151 L150 L149 L148 | L201 L206 L205 L204 L203 L202 | L213 L218 L217 L216 L215 L214 | L219 L224 L223 L222 L221 L220 | L225 L230 L229 L228 L227 L226 | L231 L236 L235 L234 L233 L232 | L243 L248 L247 L246 L245 L244 | L273 L278 L277 L276 L275 L274 | L285 L290 L289 L288 L287 L286 | L291 L296 L295 L294 L293 L292 | L297 L302 L301 L300 L299 L298 | L303 L308 L307 L306 L305 L304 | L309 L314 L313 L312 L311 L310 | L315 L320 L319 L318 L317 L316 | L321 L326 L325 L324 L323 L322 | L327 L332 L331 L330 L329 L328 | L339 L344 L343 L342 L341 L340 | L363 L368 L367 L366 L365 L364 | L369 L374 L373 L372 L371 L370 | L381 L386 L385 L384 L383 L382 | L387 L392 L391 L390 L389 L388 | L393 L398 L397 L396 L395 L394 | L399 L404 L403 L402 L401 L400 | L405 L410 L409 L408 L407 L406 | L411 L416 L415 L414 L413 L412 | L423 L428 L427 L426 L425 L424 | L435 L440 L439 L438 L437 L436 | L453 L458 L457 L456 L455 L454 | L459 L464 L463 L462 L461 L460 | L465 L470 L469 L468 L467 L466 | L471 L476 L475 L474 L473 L472 | L477 L482 L481 L480 L479 L478 | L483 L488 L487 L486 L485 L484 | L489 L494 L493 L492 L491 L490 | L495 L500 L499 L498 L497 L496 | L507 L512 L511 L510 L509 L508 | L519 L524 L523 L522 L521 L520 | L543 L548 L547 L546 L545 L544 | L549 L554 L553 L552 L551 L550 | L555 L560 L559 L558 L557 L556 | L561 L566 L565 L564 L563 L562 | L567 L572 L571 L570 L569 L568 | L573 L578 L577 L576 L575 L574 | L579 L584 L583 L582 L581 L580 | L591 L596 L595 L594 L593 L592 | L603 L608 L607 L606 L605 L604 | L615 L620 L619 L618 L617 L616 | L633 L638 L637 L636 L635 L634 | L639 L644 L643 L642 L641 L640 | L645 L650 L649 L648 L647 L646 | L651 L656 L655 L654 L653 L652 | L657 L662 L661 L660 L659 L658 | L663 L668 L667 L666 L665 L664 | L675 L680 L679 L678 L677 L676 | L687 L692 L691 L690 L689 L688 | L699 L704 L703 L702 L701 L700 | L723 L728 L727 L726 L725 L724 | L729 L734 L733 L732 L731 L730 | L735 L740 L739 L738 L737 L736 | L741 L746 L745 L744 L743 L742 | L747 L752 L751 L750 L749 L748 | L759 L764 L763 L762 L761 L760 | L771 L776 L775 L774 L773 L772 | L783 L788 L787 L786 L785 L784 | L795 L800 L799 L798 L797 L796 | L813 L818 L817 L816 L815 L814 | L819 L824 L823 L822 L821 L820 | L831 L836 L835 L834 L833 L832 | L843 L848 L847 L846 L845 L844 | L855 L860 L859 L858 L857 L856 | L867 L872 L871 L870 L869 L868 | L903 L908 L907 L906 L905 L904 | L915 L920 L919 L918 L917 L916 | L927 L932 L931 L930 L929 L928 | L939 L944 L943 L942 L941 L940 | L951 L956 L955 L954 L953 L952 | L963 L968 L967 L966 L965 L964 | L1011 L1016 L1015 L1014 L1013 L1012 | L1023 L1028 L1027 L1026 L1025 L1024 | L1035 L1040 L1039 L1038 L1037 L1036 | L1107 L1112 L1111 L1110 L1109 L1108 | L1119 L1124 L1123 L1122 L1121 L1120 | L1131 L1136 L1135 L1134 L1133 L1132
sketch "Sketch17" plane through (0, 0, 20) normal (0, 0, -1) x (-1, 0, 0)
  circle A0 centre (-50.3, 0) radius 1.45
  circle A1 centre (0, 0) radius 47.5 projected
  dimension "d96" = 2.9
  dimension "d97" = 1.35
  constraints: 1 centre point, 1 horizontal alignment
  measures "d96" diameter of A0
extrude "Extrusion13" cut sketch "Sketch17" against normal blind 5 contours A0
pattern_circular "Circular Pattern3" count 6 over 360 about axis through (0, 0, 0) along (0, 0, 1) of "Extrusion13"
sketch "Sketch18" plane through (0, 0, 40) normal (0, 0, 1) x (1, 0, 0)
  line L0 (0, 0) -> (35.5675, -35.5675)
  line L1 (0, 0) -> (50.3, 0) construction
  circle A0 centre (35.5675, -35.5675) radius 1.45
  circle A1 centre (0, 0) radius 47.5 projected
  dimension "d103" = 45
  dimension "d104" = 2.9
  dimension "d105" = 1.35
  constraints: 4 end point, 1 centre point, 1 coincident, 1 equal length, 1 horizontal
  measures "d103" angle of L0 L1
  measures "d104" diameter of A0
extrude "Extrusion14" cut sketch "Sketch18" against normal blind 5 contours A0
pattern_circular "Circular Pattern4" count 6 over 360 about axis through (0, 0, 0) along (0, 0, 1) of "Extrusion14"
sketch "Sketch19" plane through (0, 0, 10) normal (0, 0, 1) x (1, 0, 0)
  circle A0 centre (0, 0) radius 9.4
  circle A1 centre (-7, 0) radius 2.1
  circle A2 centre (0, -7) radius 2.1
  circle A3 centre (7, 0) radius 2.1
  circle A4 centre (0, 7) radius 2.1
  circle A5 centre (0, 0) radius 3
  dimension "d120" = 18.8
  dimension "d121" = 4.2
  dimension "d122" = 7
  dimension "d123" = 360
  dimension "d124" = 7
  dimension "d125" = 6
  constraints: 6 centre point, 4 coincident, 9 other
  measures "d120" diameter of A0
  measures "d121" diameter of A1
  measures "d122" distance of point (0, 0) A1.centre
  measures "d124" horizontal distance of A2.centre A1.centre
  measures "d125" diameter of A5
extrude "Extrusion15" cut sketch "Sketch19" against normal blind 50 contours A5
hole "Hole2" at (0, 7, 10) at (0, -7, 10) at (7, 0, 10) at (-7, 0, 10) direction (0, 0, -1) diameter 4 depth 7 countersink diameter 4.2 countersink angle 90
body "Solid2"
